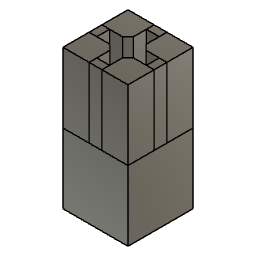
cross_hole (Autodesk Fusion 360 design; units mm, degrees)
Autodesk Fusion 360 part; units mm, degrees
sketch "Sketch1" plane through (0, 0, 0) normal (0, 0, 1) x (1, 0, 0)
  line L0 (13.95, -13.95) -> (-13.95, -13.95)
  line L1 (-13.95, -13.95) -> (-13.95, 13.95)
  line L2 (-13.95, 13.95) -> (13.95, 13.95)
  line L3 (13.95, 13.95) -> (13.95, -13.95)
  line L4 (13.95, -13.95) -> (-13.95, 13.95) construction
  line L5 (-13.95, -13.95) -> (13.95, 13.95) construction
  dimension "d1" = 27.9
  dimension "d2" = 27.9
  constraint horizontal L0
  constraint perpendicular L0 L1
  constraint parallel L0 L2
  constraint parallel L1 L3
  constraint coincident L4 origin
  constraint coincident L5 origin
  measures "d1" distance of L1.end L2.end
  measures "d2" distance of L0.end L1.end
extrude "Extrude1" add sketch "Sketch1" against normal blind 30 makes body 1
sketch "Sketch2" plane through (0, 0, 0) normal (0, 0, 1) x (-1, 0, 0)
  line L0 (-13.95, -13.95) -> (13.95, -13.95)
  line L1 (13.95, -13.95) -> (13.95, 13.95)
  line L2 (13.95, 13.95) -> (-13.95, 13.95)
  line L3 (-13.95, 13.95) -> (-13.95, -13.95)
  line L4 (13.95, -13.95) -> (2.75, -13.95)
  line L5 (2.75, -13.95) -> (2.75, -5.05)
  line L6 (5.05, -2.75) -> (13.95, -2.75)
  line L7 (13.95, -2.75) -> (13.95, -13.95)
  line L8 (5.05, -2.75) -> (2.75, -5.05)
  dimension "d5" = 11.2
  dimension "d6" = 11.2
  dimension "d22" = 2.3
  constraint horizontal L4
  constraint vertical L5
  constraint horizontal L6
  constraint vertical L7
  constraint coincident L0.end L1.start
  measures "d5" distance of L0.end L4.end
  measures "d6" distance of L0.end L6.end
  measures "d22" distance of L5 L6.start
extrude "Extrude2" add sketch "Sketch2" along normal blind 30 separate body contours L0 L1 L4 L5 L6 L7 L8 makes body 2
mirror "Mirror1" about plane through (0, 0, 0) normal (0, 1, 0) of bodies 2 makes body 3
mirror "Mirror2" about plane through (0, 0, 0) normal (1, 0, 0) of bodies 3 2 makes body 4 at (6.4833, 13.95, 20) makes body 5 at (6.4833, -13.95, 20)
sketch "Sketch3" plane through (0, 0, 0) normal (0, 0, 1) x (-1, 0, 0)
  line L0 (-13.95, -13.95) -> (13.95, -13.95)
  line L1 (13.95, -13.95) -> (13.95, 13.95)
  line L2 (13.95, 13.95) -> (-13.95, 13.95)
  line L3 (-13.95, 13.95) -> (-13.95, -13.95)
  line L4 (13.95, -2.75) -> (10.65, -2.75)
  line L5 (10.65, -2.75) -> (10.65, 2.75)
  line L6 (10.65, 2.75) -> (13.95, 2.75)
  line L7 (13.95, 2.75) -> (13.95, -2.75)
  line L8 (13.95, 2.75) -> (5.05, 2.75)
  line L9 (13.95, -2.75) -> (5.05, -2.75)
  dimension "d17" = 3.3
  constraint horizontal L4
  constraint vertical L5
  constraint horizontal L6
  constraint vertical L7
  constraint coincident L1 L4.start
  constraint coincident L5.end L8
  constraint coincident L4.end L9
  measures "d17" distance of L5 L7
extrude "Extrude3" add sketch "Sketch3" along normal blind 30 separate body contours L1 L4 L5 L6 L7 L8 L9 makes body 6
pattern_circular "C-Pattern1" count 4 over 360 about axis through (0, 0, 1.75) along (0, 0, 1) of bodies 6 makes body 7 at (-0.9167, -13.95, 10) makes body 8 at (13.95, -0.9167, 10) makes body 9 at (0.9167, 13.95, 10)
move_body "Move1" bodies 8 6 4 5 9 7 1 3 2 to x (1, 0, 0) y (0, 1, 0) z (0, 0, 1) at (0, 0, -30)
